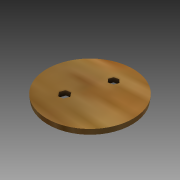
# Autodesk Inventor part: BottomHolder
Saved by Autodesk Inventor 2014 (Build 180170000, 170)
## iProperties
Created: 2013-12-17
Part Number: BottomHolder
Material: Generic
Document SubType Name: Modeling
Designer: blacki
Density: 1 g/cm^3
Appearance: Plywood - New
Author: blacki
Autodesk Inventor part; units mm, degrees
ref_plane "YZ Plane" through (0, 0, 0) normal (1, 0, 0) x (0, 1, 0)
ref_plane "XZ Plane" through (0, 0, 0) normal (0, 1, 0) x (-1, 0, 0)
ref_plane "XY Plane" through (0, 0, 0) normal (0, 0, 1) x (1, 0, 0)
sketch "Sketch1" plane through (0, 0, 0) normal (0, 0, 1) x (1, 0, 0)
  circle A0 centre (0, 0) radius 27.5
  dimension "d0" = 55
  constraints: 1 centre point, 1 coincident
  measures "d0" diameter of A0
extrude "Extrusion1" add sketch "Sketch1" along normal blind 3
sketch "Sketch2" plane through (0, 0, 0) normal (0, 0, -1) x (-1, 0, 0)
  circle A0 centre (-4.1302, 11.7979) radius 1.5 construction
  circle A1 centre (4.1302, -11.7979) radius 1.5 construction
  line L0 (-2.0593, 14.2051) -> (-1.0101, 11.208)
  line L1 (-1.0101, 11.208) -> (-3.081, 8.8009)
  line L2 (-3.081, 8.8009) -> (-6.2011, 9.3908)
  line L3 (-6.2011, 9.3908) -> (-7.2504, 12.3878)
  line L4 (-7.2504, 12.3878) -> (-5.1794, 14.795)
  line L5 (-5.1794, 14.795) -> (-2.0593, 14.2051)
  line L6 (6.2011, -9.3908) -> (7.2504, -12.3878)
  line L7 (7.2504, -12.3878) -> (5.1794, -14.795)
  line L8 (5.1794, -14.795) -> (2.0593, -14.2051)
  line L9 (2.0593, -14.2051) -> (1.0101, -11.208)
  line L10 (1.0101, -11.208) -> (3.081, -8.8009)
  line L11 (3.081, -8.8009) -> (6.2011, -9.3908)
  dimension "d7" = 5.5
  dimension "d8" = 5.5
  constraints: 24 end point, 2 coincident, 1 collinear, 26 other
  measures "d7" distance between parallel lines of L0 L3
  measures "d8" distance between parallel lines of L6 L9
extrude "Extrusion2" cut sketch "Sketch2" against normal up to next
equation "\"d8\" = d7"
body "Solid1"
